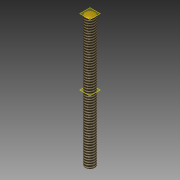
# Autodesk Inventor part: Motor_Thread
Saved by Autodesk Inventor 2011 SP2 (Build 150309200, 309)
## iProperties
Created: 2010-11-19
Part Number: Motor_Thread
Document SubType Name: Modeling
Designer: sungwook
Density: 8.47 g/cm^3
Material: Brass, Soft Yellow
Mass: 0.0838835 g
Surface Area: 0.398297 cm^2
Volume: 0.0099036 cm^3
Author: sungwook
Autodesk Inventor part; units mm, degrees
ref_plane "YZ Plane" through (0, 0, 0) normal (1, 0, 0) x (0, 1, 0)
ref_plane "XZ Plane" through (0, 0, 0) normal (0, 1, 0) x (-1, 0, 0)
sketch "Sketch1" plane through (0, 0, 0) normal (0, 0, 1) x (1, 0, 0)
  circle A0 centre (0, 0) radius 0.515
  dimension "d0" = 1.03
  constraints: 1 centre point, 1 coincident
  measures "d0" diameter of A0
extrude "Extrusion1" add sketch "Sketch1" along normal blind 14.5
thread "Thread1" size "110-102 UNM" class "2A" standard "ANSI Unified Screw Threads" full length
sketch "Sketch2" plane through (0, 0, 0) normal (1, 0, 0) x (0, 1, 0)
  line L0 (-0.515, 14.5) -> (0.515, 14.5) projected
  line L1 (-0.515, 0) -> (-0.515, 14.5) projected
  line L2 (0.515, 0) -> (0.515, 14.5) projected
  arc A0 (0, 0) -> (0.515, 0.1161) centre (0, 1.2) ccw
  line L3 (-0.515, 0) -> (0.515, 0) projected
  line L4 (0.515, 0.1161) -> (0.515, 0)
  line L5 (0, 0) -> (0.515, 0)
  line L6 (0, -2.7344) -> (0, 16.2057) projected
  point P0 (0, 0)
  point P1 (0, 0)
  constraints: 4 end point, 2 perpendicular, 2 point on circle, 2 tangent, 1 centre point, 1 coincident, 1 midpoint, 1 point on line, 1 vertical alignment
revolve "Revolution1" cut sketch "Sketch2" angle 360 about axis through (0, 0, -10) along (0, 0, 1) contours A0 L2 L3
ref_plane "Work Plane_Mid" through (0, 0, 7.25) normal (0, 0, 1) x (1, 0, 0)
mirror "Mirror1" about plane through (0, 0, 7.25) normal (0, 0, 1) of "Revolution1"
ref_plane "Work Plane4" through (0, 0, 14.5) normal (0, 0, 1) x (1, 0, 0)
equation "\"d10\" = 0.5 * d1"
equation "\"d11\" = d1"
equation "\"d1\" = 14.5"
body "Solid1"
